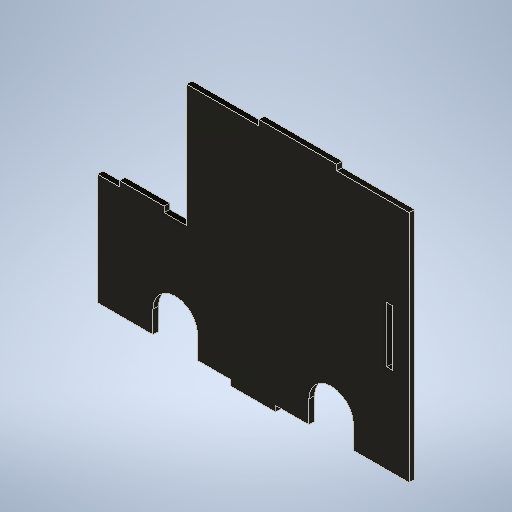
# Autodesk Inventor part: side
Saved by Autodesk Inventor 2025.3 (Build 293356030, 356C)
## iProperties
Created: 2026-06-26
Part Number: side
Material: Generic
Document SubType Name: Modeling
Designer: user
Density: 1 g/cm^3
Appearance: Gunmetal
Author: user
Autodesk Inventor part; units mm, degrees
ref_plane "YZ Plane" through (0, 0, 0) normal (1, 0, 0) x (0, 1, 0)
ref_plane "XZ Plane" through (0, 0, 0) normal (0, 1, 0) x (-1, 0, 0)
ref_plane "XY Plane" through (0, 0, 0) normal (0, 0, 1) x (1, 0, 0)
sketch "Sketch1" plane through (0, 0, 0) normal (0, 0, 1) x (1, 0, 0)
  line L0 (0, 0) -> (0, 100)
  line L1 (0, 100) -> (80, 100)
  line L2 (80, 100) -> (80, 210)
  line L3 (80, 210) -> (280, 210)
  line L4 (280, 210) -> (280, 0)
  line L5 (0, 0) -> (50, 0)
  line L6 (50, 0) -> (50, 20)
  arc A0 (90, 20) -> (50, 20) centre (70, 20) ccw
  line L7 (90, 20) -> (90, 0)
  line L8 (140, 0) -> (140, 210) construction
  line L9 (90, 0) -> (140, 0)
  line L10 (280, 0) -> (230, 0)
  line L11 (230, 0) -> (230, 20)
  arc A1 (230, 20) -> (190, 20) centre (210, 20) ccw
  line L12 (190, 20) -> (190, 0)
  line L13 (190, 0) -> (140, 0)
  line L14 (145, 210) -> (215, 210)
  line L15 (215, 210) -> (215, 215)
  line L16 (215, 215) -> (145, 215)
  line L17 (145, 215) -> (145, 210)
  line L18 (265, 80) -> (260, 80)
  line L19 (260, 80) -> (260, 130)
  line L20 (260, 130) -> (265, 130)
  line L21 (265, 130) -> (265, 80)
  line L22 (10, 20) -> (15, 20)
  line L23 (15, 20) -> (15, 60)
  line L24 (15, 60) -> (10, 60)
  line L25 (10, 60) -> (10, 20)
  line L26 (20, 100) -> (60, 100)
  line L27 (60, 100) -> (60, 105)
  line L28 (60, 105) -> (20, 105)
  line L29 (20, 105) -> (20, 100)
  line L30 (160, 0) -> (160, -5)
  line L31 (160, -5) -> (120, -5)
  line L32 (120, -5) -> (120, 0)
  dimension "d0" = 100
  dimension "d1" = 80
  dimension "d2" = 110
  dimension "d3" = 200
  dimension "d4" = 50
  dimension "d5" = 20
  dimension "d6" = 40
  dimension "d7" = 70
  dimension "d8" = 5
  dimension "d9" = 5
  dimension "d10" = 50
  dimension "d12" = 50
  dimension "d13" = 5
  dimension "d14" = 40
  dimension "d17" = 40
  dimension "d18" = 5
  dimension "d19" = 40
  dimension "d20" = 5
  dimension "d21" = 20
  constraints: 66 end point, 12 perpendicular, 9 parallel, 6 horizontal, 5 point on line, 5 symmetric about line, 4 point on circle, 2 centre point, 2 tangent, 2 vertical, 1 other
  measures "d0" distance of L0.start L0.end
  measures "d1" distance of L0.end L1.end
  measures "d2" distance of L1.end L2.end
  measures "d3" distance of L2.end L3.end
  measures "d4" distance of L0.start L5.end
  measures "d5" distance of L5.end L6.end
  measures "d6" distance of L6.end L7.start
  measures "d7" distance of L16.end L15.end
  measures "d8" distance of L15.end L14.end
  measures "d9" distance of L19.end L20.end
  measures "d10" distance of L18.end L19.end
  measures "d12" distance between parallel lines of L4 L11
  measures "d13" distance of L24.end L23.end
  measures "d14" distance of L23.end L22.end
  measures "d17" distance of L28.end L27.end
  measures "d18" distance of L27.end L26.end
  measures "d19" distance of L30.end L31.end
  measures "d20" distance of L30.start L30.end
  measures "d21" distance between parallel lines of L32 L8
extrude "Extrusion1" add sketch "Sketch1" along normal blind 5 contours L0 L1 L2 L3 L4 L10 L11 A1 L12 L13 L9 L7 A0 L6 L5 | L29 L28 L27 L1 | L9 L13 L30 L31 L32 | L17 L16 L15 L3 | L25 L24 L23 L22
body "Solid1"
